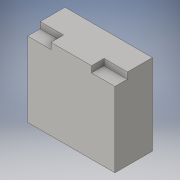
# Autodesk Inventor part: Battery
Saved by Autodesk Inventor 2016 SP2 (Build 200236200, 236)
## iProperties
Created: 2018-01-09
Part Number: Battery
Material: Generic
Document SubType Name: Modeling
Designer: CAD
Density: 1 g/cm^3
Appearance: Default
Author: CAD
Autodesk Inventor part; units mm, degrees
ref_plane "YZ Plane" through (0, 0, 0) normal (1, 0, 0) x (0, 1, 0)
ref_plane "XZ Plane" through (0, 0, 0) normal (0, 1, 0) x (-1, 0, 0)
ref_plane "XY Plane" through (0, 0, 0) normal (0, 0, 1) x (1, 0, 0)
sketch "Sketch1" plane through (0, 0, 0) normal (0, 1, 0) x (-1, 0, 0)
  line L0 (0, 0) -> (-177.8, 0)
  line L1 (-177.8, 0) -> (-177.8, -76.2)
  line L2 (-177.8, -76.2) -> (0, -76.2)
  line L3 (0, -76.2) -> (0, 0)
  dimension "d0" = 177.8
  dimension "d1" = 76.2
  constraints: 8 end point, 3 perpendicular, 1 horizontal
  measures "d0" distance of L0.start L0.end
  measures "d1" distance of L0.end L1.end
extrude "Extrusion1" add sketch "Sketch1" along normal blind 165.1
sketch "Sketch2" plane through (0, 165.1, 0) normal (0, 1, 0) x (1, 0, 0)
  line L0 (177.8, 25.4) -> (130.175, 25.4)
  line L1 (130.175, 25.4) -> (130.175, 0)
  line L2 (0, 25.4) -> (47.625, 25.4)
  line L3 (47.625, 25.4) -> (47.625, 0)
  line L4 (0, 0) -> (177.8, 0) projected
  line L5 (0, 76.2) -> (0, 0) projected
  line L6 (177.8, 0) -> (177.8, 76.2) projected
  line L7 (0, 25.4) -> (0, 0)
  line L8 (0, 0) -> (47.625, 0)
  line L9 (130.175, 0) -> (177.8, 0)
  line L10 (177.8, 25.4) -> (177.8, 0)
  dimension "d4" = 47.625
  dimension "d5" = 47.625
  dimension "d6" = 25.4
  dimension "d7" = 25.4
  constraints: 16 end point, 3 collinear, 3 perpendicular, 3 point on line, 1 horizontal
  measures "d4" distance between parallel lines of L5 L3
  measures "d5" distance between parallel lines of L6 L1
  measures "d6" distance between parallel lines of L4 L2
  measures "d7" distance between parallel lines of L4 L0
extrude "Extrusion2" cut sketch "Sketch2" against normal blind 12.7
body "Solid1"
